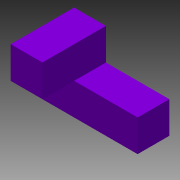
# Autodesk Inventor part: Part 2.1
Saved by Autodesk Inventor 2013 (Build 170138000, 138)
## iProperties
Created: 2013-11-13
Part Number: Part 2.1
Material: Generic
Document SubType Name: Modeling
Designer: s601298
Density: 1 g/cm^3
Mass: 34.5665 g
Surface Area: 79.8385 cm^2
Volume: 34.5665 cm^3
Author: s601298
Autodesk Inventor part; units mm, degrees
ref_plane "YZ Plane" through (0, 0, 0) normal (1, 0, 0) x (0, 1, 0)
ref_plane "XZ Plane" through (0, 0, 0) normal (0, 1, 0) x (-1, 0, 0)
ref_plane "XY Plane" through (0, 0, 0) normal (0, 0, 1) x (1, 0, 0)
sketch "Sketch1" plane through (0, 0, 0) normal (0, 0, 1) x (1, 0, 0)
  line L0 (-18.0321, 15.2691) -> (39.1179, 15.2691)
  line L1 (39.1179, 15.2691) -> (39.1179, -3.7809)
  line L2 (39.1179, -3.7809) -> (-18.0321, -3.7809)
  line L3 (-18.0321, -3.7809) -> (-18.0321, 15.2691)
  point P0 (0, 0)
  dimension "d0" = 57.15
  dimension "d2" = 19.05
  constraints: 8 end point, 2 parallel, 1 horizontal, 1 perpendicular
  measures "d0" distance of L0.start L0.end
  measures "d2" distance of L2.end L0.start
extrude "Extrusion1" add sketch "Sketch1" along normal blind 19.05
sketch "Sketch2" plane through (-18.0321, 15.2691, 0) normal (0, 1, 0) x (1, 0, 0)
  line L0 (0, 0) -> (19.05, 0)
  line L1 (19.05, 0) -> (19.05, -38.1)
  line L2 (19.05, -38.1) -> (0, -38.1)
  line L3 (0, -38.1) -> (0, 0)
  point P0 (18.0321, 0)
  dimension "d5" = 19.05
  dimension "d6" = 38.1
  constraints: 8 end point, 2 parallel, 1 horizontal, 1 perpendicular
  measures "d5" distance of L1.end L2.end
  measures "d6" distance of L0.end L1.end
extrude "Extrusion2" add sketch "Sketch2" along normal blind 19.05
body "Solid1"
